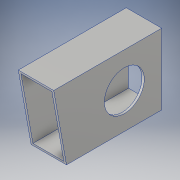
# Autodesk Inventor part: ARM_029_BottomIntakeSide
Saved by Autodesk Inventor 2018 (Build 220112000, 112)
## iProperties
Created: 2020-02-04
Part Number: ARM_029_BottomIntakeSide
Material: Aluminum 6061
Document SubType Name: Modeling
Designer: 22turnmaxw
Density: 2.7 g/cm^3
Appearance: Aluminum - Flat
Author: 22turnmaxw
Autodesk Inventor part; units mm, degrees
ref_plane "YZ Plane" through (0, 0, 0) normal (1, 0, 0) x (0, 1, 0)
ref_plane "XZ Plane" through (0, 0, 0) normal (0, 1, 0) x (-1, 0, 0)
ref_plane "XY Plane" through (0, 0, 0) normal (0, 0, 1) x (1, 0, 0)
sketch "Sketch1" plane through (0, 0, 0) normal (0, 0, 1) x (1, 0, 0)
  line L0 (0, 0) -> (25.4, 0)
  line L1 (25.4, 0) -> (25.4, 50.8)
  line L2 (25.4, 50.8) -> (0, 50.8)
  line L3 (0, 50.8) -> (0, 0)
  line L4 (1.5875, 1.5875) -> (23.8125, 1.5875)
  line L5 (23.8125, 1.5875) -> (23.8125, 49.2125)
  line L6 (23.8125, 49.2125) -> (1.5875, 49.2125)
  line L7 (1.5875, 49.2125) -> (1.5875, 1.5875)
  dimension "d0" = 25.4
  dimension "d1" = 50.8
  dimension "d2" = 1.5875
  constraints: 16 end point, 4 parallel, 2 perpendicular, 1 horizontal, 3 other
  measures "d0" distance of L1.end L2.end
  measures "d1" distance of L0.end L1.end
  measures "d2" distance between parallel lines of L3 L7
extrude "Extrusion1" add sketch "Sketch1" along normal blind 77.4446
sketch "Sketch2" plane through (25.4, 0, 0) normal (1, 0, 0) x (0, 0, -1)
  line L0 (0, 50.8) -> (-77.4446, 50.8) projected
  line L1 (-77.4446, 50.8) -> (-68.2676, 0)
  line L2 (-68.2676, 0) -> (-77.4446, 0)
  line L3 (0, 1.5875) -> (-77.4446, 1.5875) projected
  line L4 (-77.4446, 50.8) -> (-77.4446, 0) projected
  line L5 (-77.4446, 0) -> (-77.4446, 50.8)
  point P0 (0, 0)
  dimension "d5" = 10.24
  constraints: 6 end point, 1 collinear, 1 parallel
  measures "d5" angle of L4 L1
sketch "Sketch3" plane through (25.4, 0, 0) normal (1, 0, 0) x (0, 0, -1)
  line L0 (0, 0) -> (0, 50.8) projected
  line L1 (0, 50.8) -> (-77.4446, 50.8) projected
  line L2 (-77.4446, 0) -> (-77.4446, 50.8) projected
  point P0 (-26.797, 25.4)
  dimension "d10" = 25.4
  dimension "d21" = 50.6476
  measures "d10" distance from line of L1 point (-26.797, 25.4)
  measures "d21" distance from line of L2 point (-26.797, 25.4)
hole "Hole1" at (25.4, 25.4, 26.797) direction (-1, 0, 0) diameter 28.575 depth 25.4 tip angle 118
extrude "Extrusion3" cut sketch "Sketch2" against normal blind 25.4
body "Solid1"
